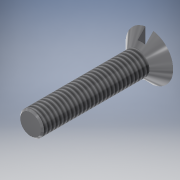
# Autodesk Inventor part: XGEN_M3_screw
Saved by Autodesk Inventor 2019 (Build 230136000, 136)
## iProperties
Created: 2007-03-09
Part Number: XGEN_M3_screw
Document SubType Name: Modeling
Designer: RBodenst
Density: 1 g/cm^3
Material: Generic
Appearance: Aluminum - Polished
Author: RBodenst
Autodesk Inventor part; units mm, degrees
ref_plane "YZ Plane" through (0, 0, 0) normal (1, 0, 0) x (0, 1, 0)
ref_plane "XZ Plane" through (0, 0, 0) normal (0, 1, 0) x (-1, 0, 0)
ref_plane "XY Plane" through (0, 0, 0) normal (0, 0, 1) x (1, 0, 0)
sketch "Sketch1" plane through (0, 0, 0) normal (0, 0, 1) x (1, 0, 0)
  line L0 (0, 0) -> (1.5, 0)
  line L1 (1.5, 0) -> (1.5, 13.5)
  line L2 (1.5, 13.5) -> (3, 15)
  line L3 (3, 15) -> (0, 15)
  line L4 (0, 15) -> (0, 0)
  line L5 (0, -3) -> (0, 18) projected
  dimension "d2" = 1.5
  dimension "d3" = 15
  dimension "d6" = 0
  dimension "d7" = 0
  dimension "d8" = 45
  dimension "d9" = 3
  constraints: 10 end point, 2 parallel, 1 horizontal, 1 perpendicular
  measures "d2" distance of L0.start L0.end
  measures "d3" distance of L3.end L0.start
  measures "d6" distance from line of L5 L0.start
  measures "d7" distance of point (0, 0) L0.start
  measures "d8" angle of L3 L2
  measures "d9" distance of L2.end L3.end
revolve "Revolution1" add sketch "Sketch1" angle 360 about axis through (0, -10, 0) along (0, 1, 0)
sketch "Sketch2" plane through (0, 15, 0) normal (0, 1, 0) x (1, 0, 0)
  circle A0 centre (0, 0) radius 3 projected
  line L0 (-0.5, 5.0208) -> (0.5, 5.0208)
  line L1 (0.5, 5.0208) -> (0.5, -4.425)
  line L2 (0.5, -4.425) -> (-0.5, -4.425)
  line L3 (-0.5, -4.425) -> (-0.5, 5.0208)
  dimension "d10" = 1
  dimension "d11" = 0.5
  constraints: 8 end point, 2 parallel, 1 horizontal, 1 perpendicular
  measures "d10" distance of L1.end L2.end
  measures "d11" horizontal distance of A0.centre L2.end
extrude "Extrusion1" cut sketch "Sketch2" against normal blind 1 contours L1 A0 L3 | A0 L3 L0 L1 | L1 L2 L3 A0
thread "Thread2" size "M3x0.5" class "6g" standard "ANSI Metric M Profile" full length
chamfer "Chamfer1" distance 0.2 angle 45 1 edges at (-1.5, 0, 0)
equation "\"d11\" = 0.5 * d10"
body "Solid1"
